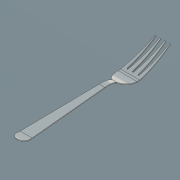
# Autodesk Inventor part: eating fork
Saved by Autodesk Inventor 2020 (Build 240168000, 168)
## iProperties
Created: 2019-12-06
Part Number: eating fork
Material: Iron, Cast
Document SubType Name: Modeling
Designer: User
Density: 7.15 g/cm^3
Appearance: Machined - Aluminum
Author: User
Autodesk Inventor part; units mm, degrees
ref_plane "YZ Plane" through (0, 0, 0) normal (1, 0, 0) x (0, 1, 0)
ref_plane "XZ Plane" through (0, 0, 0) normal (0, 1, 0) x (-1, 0, 0)
ref_plane "XY Plane" through (0, 0, 0) normal (0, 0, 1) x (1, 0, 0)
sketch "Sketch1" plane through (0, 0, 0) normal (0, 1, 0) x (-1, 0, 0)
  line L0 (0, 0) -> (25, 0)
  line L1 (25, 0) -> (25, -200)
  line L2 (25, -200) -> (0, -200)
  line L3 (0, -200) -> (0, 0)
  dimension "d0" = 25
  dimension "d1" = 200
  constraints: 8 end point, 2 parallel, 1 horizontal, 1 perpendicular
  measures "d0" distance of L1.end L2.end
  measures "d1" distance of L0.end L1.end
extrude "Extrusion1" add sketch "Sketch1" along normal blind 20
sketch "Sketch2" plane through (0, 20, 0) normal (0, 1, 0) x (1, 0, 0)
  line L0 (0, 200) -> (-25, 200) projected
  line L1 (-2.5, 200) -> (-22.5, 200)
  line L2 (-22.5, 200) -> (-22.5, 135)
  line L3 (-22.5, 135) -> (-2.5, 135)
  line L4 (-2.5, 135) -> (-2.5, 200)
  line L5 (-25, 200) -> (-25, 0) projected
  line L6 (-19.7046, 160) -> (-22.5, 160)
  line L7 (0, 0) -> (0, 200) projected
  line L8 (0, 160) -> (-2.5, 200)
  line L9 (-25, 160) -> (-22.5, 200)
  line L10 (-25, 160) -> (-25, 156)
  line L11 (0, 160) -> (0, 156)
  line L12 (-15.5, 135) -> (-9.5, 135)
  line L13 (-9.5, 135) -> (-9.5, 149.6928)
  line L14 (-9.5, 149.6928) -> (-15.5, 149.6928)
  line L15 (-15.5, 149.6928) -> (-15.5, 135)
  line L16 (-12.5, 200) -> (-12.5, 135)
  arc A0 (-9.1086, 135.3101) -> (0, 156) centre (-24.623, 154.4902) ccw
  arc A1 (-25, 156) -> (-15.9105, 135.3093) centre (-1.5252, 153.9707) ccw
  line L17 (-22.5, 200) -> (-21.5, 200)
  line L18 (-21.5, 200) -> (-20.5183, 160.7313)
  line L19 (-19.7685, 160) -> (-19, 160)
  line L20 (-18.956, 160.7032) -> (-16.5, 200)
  line L21 (-2.5, 200) -> (-3.5, 200)
  line L22 (-3.5, 200) -> (-4.4817, 160.7313)
  line L23 (-5.2315, 160) -> (-5.2954, 160)
  line L24 (-6.044, 160.7032) -> (-8.5, 200)
  line L25 (-16.5, 200) -> (-15, 200)
  line L26 (-15, 200) -> (-13.2814, 160.7172)
  line L27 (-12.5321, 160) -> (-12.4679, 160)
  line L28 (-8.5, 200) -> (-10, 200)
  line L29 (-10, 200) -> (-11.7186, 160.7172)
  line L30 (-11.75, 160) -> (-13.25, 160)
  arc A2 (-5.2315, 160) -> (-4.4817, 160.7313) centre (-5.2315, 160.75) ccw
  arc A3 (-6.044, 160.7032) -> (-5.2954, 160) centre (-5.2954, 160.75) ccw
  arc A4 (-19.7046, 160) -> (-18.956, 160.7032) centre (-19.7046, 160.75) ccw
  arc A5 (-20.5183, 160.7313) -> (-19.7685, 160) centre (-19.7685, 160.75) ccw
  arc A6 (-13.2814, 160.7172) -> (-12.5321, 160) centre (-12.5321, 160.75) ccw
  arc A7 (-12.4679, 160) -> (-11.7186, 160.7172) centre (-12.4679, 160.75) ccw
  line L31 (-9.5, 135) -> (-15.5, 135)
  line L32 (-15.5, 135) -> (-15.5, 15)
  line L33 (-15.5, 15) -> (-9.5, 15)
  line L34 (-9.5, 15) -> (-9.5, 135)
  line L35 (-4.5, 15) -> (-20.5, 15)
  line L36 (-4.5, 15) -> (-9.4788, 134.491)
  line L37 (-15.5218, 134.4757) -> (-20.5, 15)
  arc A8 (-15.5218, 134.4757) -> (-15.9105, 135.3093) centre (-16.521, 134.5173) ccw
  arc A9 (-9.1086, 135.3101) -> (-9.4788, 134.491) centre (-8.4797, 134.5326) ccw
  circle A10 centre (-12.5, 15) radius 8
  line L38 (0, 152.9803) -> (0, 0)
  line L39 (-25, 0) -> (0, 0) projected
  line L40 (0, 0) -> (-25, 0)
  line L41 (-25, 0) -> (-25, 151.9415)
  point P0 (-2.5, 160)
  point P1 (-20.5, 160)
  point P2 (-4.5, 160)
  point P3 (-6, 160)
  point P4 (-11.75, 160)
  point P5 (-4.5277, 15.6655)
  point P6 (-20.4723, 15.6655)
  dimension "d4" = 20
  dimension "d5" = 2.5
  dimension "d6" = 65
  dimension "d7" = 40
  dimension "d8" = 4
  dimension "d9" = 6
  dimension "d10" = 3
  dimension "d11" = 1
  dimension "d12" = 1.5
  dimension "d13" = 5
  dimension "d14" = 1.5
  dimension "d15" = 5.75
  dimension "d18" = 1.5
  dimension "d19" = 1.5
  dimension "d20" = 5.75
  dimension "d21" = 5
  dimension "d22" = 0.75
  dimension "d23" = 0.75
  dimension "d24" = 0.75
  dimension "d25" = 0.75
  dimension "d26" = 0.75
  dimension "d27" = 6
  dimension "d28" = 120
  dimension "d29" = 16
  dimension "d30" = 5
  dimension "d31" = 1
  dimension "d32" = 1
  constraints: 76 end point, 33 point on line, 24 point on circle, 16 tangent, 10 centre point, 6 parallel, 4 horizontal, 4 perpendicular, 4 symmetric about line, 3 collinear, 3 midpoint, 1 equal radius, 3 other
  measures "d4" distance of L2.end L3.end
  measures "d5" distance between parallel lines of L5 L2
  measures "d6" distance of L3.end L1.start
  measures "d7" distance between parallel lines of L0 L6
  measures "d8" distance of L9.start L10.end
  measures "d9" distance of L13.end L14.end
  measures "d10" distance between parallel lines of L15 L16
  measures "d11" distance of L1.end L17.end
  measures "d12" distance of point (-20.5, 160) L19.end
  measures "d13" distance of L17.end L20.end
  measures "d14" distance of L20.end L25.end
  measures "d15" distance of L19.end L30.end
  measures "d18" distance of L24.end L28.end
  measures "d19" distance of L30.end L30.start
  measures "d20" distance of point (-11.75, 160) point (-6, 160)
  measures "d21" distance of L24.end L22.start
  measures "d22" radius of A2
  measures "d23" radius of A3
  measures "d24" radius of A4
  measures "d25" radius of A6
  measures "d26" radius of A7
  measures "d27" distance of L33.end L32.end
  measures "d28" distance of L32.end L31.end
  measures "d29" distance of L35.start L35.end
  measures "d30" distance of L33.end L35.start
  measures "d31" radius of A8
  measures "d32" radius of A9
extrude "Extrusion2" cut sketch "Sketch2" against normal blind 21 contours L7 L8 L0 | L22 A2 L23 A3 L24 L0 | A0 L7 L39 L5 A1 L2 L3 A8 L37 A10 L36 A9 L4 | L4 L3 A9 A0 | L29 A7 L27 L16 L0 | L16 L27 A6 L26 L0 | L20 A4 L6 A5 L18 L0 | A1 A8 L3 L2 | L5 L0 L9
sketch "Sketch3" plane through (0, 0, 0) normal (1, 0, 0) x (0, 1, 0)
  line L0 (0, -134.491) -> (0, -15.6655) projected
  line L1 (20, -134.491) -> (0, -134.491) projected
  line L2 (20, -15.6655) -> (20, -134.491) projected
  line L3 (20, -15.6655) -> (0, -15.6655) projected
  line L4 (0, -15.6655) -> (0, -15.6655) projected
  line L5 (20, -15.6655) -> (0, -15.6655) projected
  line L6 (20, -15.6655) -> (20, -15.6655) projected
  line L7 (20, -15.6655) -> (0, -15.6655) projected
  line L8 (0, -135.3101) -> (0, -134.491) projected
  line L9 (20, -135.3101) -> (0, -135.3101) projected
  line L10 (20, -134.491) -> (20, -135.3101) projected
  line L11 (20, -134.491) -> (0, -134.491) projected
  line L12 (0, -152.9803) -> (0, -135.3101) projected
  line L13 (20, -152.9803) -> (0, -152.9803) projected
  line L14 (20, -135.3101) -> (20, -152.9803) projected
  line L15 (20, -135.3101) -> (0, -135.3101) projected
  line L16 (0, -200) -> (0, -160) projected
  line L17 (20, -200) -> (0, -200) projected
  line L18 (20, -160) -> (20, -200) projected
  line L19 (0, -160) -> (20, -160) projected
  line L20 (0, -160) -> (20, -160) projected
  line L21 (20, -152.9803) -> (20, -160) projected
  line L22 (20, -152.9803) -> (0, -152.9803) projected
  line L23 (0, -152.9803) -> (0, -160) projected
  line L24 (0, -152.9803) -> (0, -160) projected
  line L25 (20, -200) -> (0, -200) projected
  arc A0 (0, -156.4902) -> (18.6798, -200) centre (126.5442, -127.9265) ccw
  arc A1 (3.1491, -135.3101) -> (0, -152.9803) centre (46.6756, -152.183) ccw
  line L26 (0, -152.9803) -> (0, -156.4902)
  arc A2 (3.1491, -135.3101) -> (5.7199, -119.3952) centre (-23.6022, -122.8238) ccw
  line L27 (5.7199, -119.3952) -> (0, -19.1705)
  line L28 (0, -134.491) -> (0, -15.6655) projected
  line L29 (0, -7) -> (20, -7) projected
  arc A3 (1.3856, -7) -> (0, -19.1705) centre (58.0851, -19.6191) ccw
  arc A4 (2.3617, -7.2172) -> (1.0002, -19.146) centre (58.0851, -19.6191) ccw
  line L30 (1.0002, -19.146) -> (6.7166, -119.3088)
  arc A5 (4.0696, -135.7023) -> (6.7166, -119.3088) centre (-23.6022, -122.8238) ccw
  arc A6 (4.0696, -135.7023) -> (1, -152.9717) centre (46.6756, -152.183) ccw
  line L31 (1, -152.9717) -> (1, -156.3785)
  arc A7 (1, -156.3785) -> (19.5113, -199.4444) centre (126.5442, -127.9265) ccw
  line L32 (1.3856, -7) -> (2.3617, -7.2172)
  line L33 (18.6798, -200) -> (19.5113, -199.4444)
  line L34 (20, -15.6655) -> (20, -7) projected
  line L35 (20, -15.6655) -> (20, -7)
  line L36 (0, -7) -> (0, -15.6655)
  point P0 (0, 0)
  point P1 (0, -15.6655)
  point P2 (18.6798, -200)
  point P3 (18.6798, -200)
  point P4 (0, -151.3856)
  dimension "d36" = 1
  constraints: 16 end point, 16 point on circle, 8 centre point, 4 point on line, 2 collinear, 1 midpoint, 1 vertical, 5 other
  measures "d36" distance between parallel lines of L27 L30
extrude "Extrusion3" cut sketch "Sketch3" against normal blind 25 contours L0 L27 A2 L1 | L1 A2 L9 L8 | L0 L3 A3 | L9 A1 L12 | L36 L29 A3 L3 | A5 L30 A4 L3 L2 L1 | L1 L10 L9 A5 | A4 L32 L29 L34 L3 | L9 L14 L13 L31 A6 A5 | L13 L21 L19 A7 L31 | A0 L19 L23 | L19 A0 L17 L16 | L18 L17 L33 A7 L19
body "Solid1"
